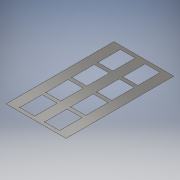
# Autodesk Inventor part: Assembly Stencil
Saved by Autodesk Inventor 2019.4 (Build 234330000, 330)
## iProperties
Created: 2021-01-11
Part Number: Assembly Stencil
Material: Stainless Steel
Document SubType Name: Modeling
Designer: caleb
Density: 8 g/cm^3
Appearance: Semi-Polished
Author: caleb
Autodesk Inventor part; units mm, degrees
ref_plane "YZ Plane" through (0, 0, 0) normal (1, 0, 0) x (0, 1, 0)
ref_plane "XZ Plane" through (0, 0, 0) normal (0, 1, 0) x (-1, 0, 0)
ref_plane "XY Plane" through (0, 0, 0) normal (0, 0, 1) x (1, 0, 0)
sketch "Sketch1" plane through (0, 0, 0) normal (0, 1, 0) x (-1, 0, 0)
  line L0 (-60, 108) -> (60, 108)
  line L1 (60, 108) -> (60, -108)
  line L2 (60, -108) -> (-60, -108)
  line L3 (-60, -108) -> (-60, 108)
  line L4 (-60, 108) -> (60, -108) construction
  line L5 (60, 108) -> (-60, -108) construction
  point P0 (0, 0)
  dimension "d0" = 216
  dimension "d1" = 120
  constraints: 12 end point, 2 midpoint, 2 parallel, 1 horizontal, 1 perpendicular
  measures "d0" distance of L0.end L1.end
  measures "d1" distance of L0.start L0.end
extrude "Extrusion1" add sketch "Sketch1" along normal blind 0.1
sketch "Sketch2" plane through (0, 0.1, 0) normal (0, 1, 0) x (1, 0, 0)
  line L0 (-40, -100.8) -> (-10.2, -100.8)
  line L1 (-10, -100.6) -> (-10, -56)
  line L2 (-10.2, -55.8) -> (-39.8, -55.8)
  line L3 (-40, -56) -> (-40, -100.8)
  line L4 (-60, -108) -> (60, -108) projected
  line L5 (-60, 108) -> (-60, -108) projected
  circle A0 centre (-40, -100.8) radius 1
  arc A1 (-39.8, -55.8) -> (-40, -56) centre (-39.8, -56) ccw
  arc A2 (-10, -56) -> (-10.2, -55.8) centre (-10.2, -56) ccw
  arc A3 (-10.2, -100.8) -> (-10, -100.6) centre (-10.2, -100.6) ccw
  line L6 (-40, -3.8) -> (-40, -48.6)
  arc A4 (-39.8, -3.6) -> (-40, -3.8) centre (-39.8, -3.8) ccw
  circle A5 centre (-40, -48.6) radius 1
  line L7 (-10.2, -3.6) -> (-39.8, -3.6)
  line L8 (-40, -48.6) -> (-10.2, -48.6)
  line L9 (-10, -48.4) -> (-10, -3.8)
  arc A6 (-10, -3.8) -> (-10.2, -3.6) centre (-10.2, -3.8) ccw
  arc A7 (-10.2, -48.6) -> (-10, -48.4) centre (-10.2, -48.4) ccw
  line L10 (-40, 48.4) -> (-40, 3.6)
  arc A8 (-39.8, 48.6) -> (-40, 48.4) centre (-39.8, 48.4) ccw
  circle A9 centre (-40, 3.6) radius 1
  line L11 (-10.2, 48.6) -> (-39.8, 48.6)
  line L12 (-40, 3.6) -> (-10.2, 3.6)
  line L13 (-10, 3.8) -> (-10, 48.4)
  arc A10 (-10, 48.4) -> (-10.2, 48.6) centre (-10.2, 48.4) ccw
  arc A11 (-10.2, 3.6) -> (-10, 3.8) centre (-10.2, 3.8) ccw
  line L14 (-40, 100.6) -> (-40, 55.8)
  arc A12 (-39.8, 100.8) -> (-40, 100.6) centre (-39.8, 100.6) ccw
  circle A13 centre (-40, 55.8) radius 1
  line L15 (-10.2, 100.8) -> (-39.8, 100.8)
  line L16 (-40, 55.8) -> (-10.2, 55.8)
  line L17 (-10, 56) -> (-10, 100.6)
  arc A14 (-10, 100.6) -> (-10.2, 100.8) centre (-10.2, 100.6) ccw
  arc A15 (-10.2, 55.8) -> (-10, 56) centre (-10.2, 56) ccw
  line L18 (10, -56) -> (10, -100.8)
  arc A16 (10.2, -55.8) -> (10, -56) centre (10.2, -56) ccw
  circle A17 centre (10, -100.8) radius 1
  line L19 (39.8, -55.8) -> (10.2, -55.8)
  line L20 (10, -100.8) -> (39.8, -100.8)
  line L21 (40, -100.6) -> (40, -56)
  arc A18 (40, -56) -> (39.8, -55.8) centre (39.8, -56) ccw
  arc A19 (39.8, -100.8) -> (40, -100.6) centre (39.8, -100.6) ccw
  line L22 (10, -3.8) -> (10, -48.6)
  arc A20 (10.2, -3.6) -> (10, -3.8) centre (10.2, -3.8) ccw
  circle A21 centre (10, -48.6) radius 1
  line L23 (39.8, -3.6) -> (10.2, -3.6)
  line L24 (10, -48.6) -> (39.8, -48.6)
  line L25 (40, -48.4) -> (40, -3.8)
  arc A22 (40, -3.8) -> (39.8, -3.6) centre (39.8, -3.8) ccw
  arc A23 (39.8, -48.6) -> (40, -48.4) centre (39.8, -48.4) ccw
  line L26 (10, 48.4) -> (10, 3.6)
  arc A24 (10.2, 48.6) -> (10, 48.4) centre (10.2, 48.4) ccw
  circle A25 centre (10, 3.6) radius 1
  line L27 (39.8, 48.6) -> (10.2, 48.6)
  line L28 (10, 3.6) -> (39.8, 3.6)
  line L29 (40, 3.8) -> (40, 48.4)
  arc A26 (40, 48.4) -> (39.8, 48.6) centre (39.8, 48.4) ccw
  arc A27 (39.8, 3.6) -> (40, 3.8) centre (39.8, 3.8) ccw
  line L30 (10, 100.6) -> (10, 55.8)
  arc A28 (10.2, 100.8) -> (10, 100.6) centre (10.2, 100.6) ccw
  circle A29 centre (10, 55.8) radius 1
  line L31 (39.8, 100.8) -> (10.2, 100.8)
  line L32 (10, 55.8) -> (39.8, 55.8)
  line L33 (40, 56) -> (40, 100.6)
  arc A30 (40, 100.6) -> (39.8, 100.8) centre (39.8, 100.6) ccw
  arc A31 (39.8, 55.8) -> (40, 56) centre (39.8, 56) ccw
  point P0 (0, 0)
  point P1 (-10, -100.8)
  point P2 (-40, -55.8)
  point P3 (-40, -3.6)
  point P4 (-10, -48.6)
  point P5 (-40, 48.6)
  point P6 (-10, 3.6)
  point P7 (-40, 100.8)
  point P8 (-10, 55.8)
  point P9 (10, -55.8)
  point P10 (40, -100.8)
  point P11 (10, -3.6)
  point P12 (40, -48.6)
  point P13 (10, 48.6)
  point P14 (40, 3.6)
  point P15 (10, 100.8)
  point P16 (40, 55.8)
  dimension "d4" = 30
  dimension "d5" = 45
  dimension "d6" = 7.2
  dimension "d7" = 20
  dimension "d8" = 2
  dimension "d9" = 0.2
  dimension "d12" = 52.2
  dimension "d15" = 50
  constraints: 64 end point, 48 point on circle, 32 centre point, 32 point on line, 8 coincident, 6 tangent, 2 equal radius, 2 horizontal, 2 parallel, 1 perpendicular, 1 vertical, 147 other
  measures "d4" distance of L0.start point (-10, -100.8)
  measures "d5" distance of point (-40, -55.8) L0.start
  measures "d6" distance between parallel lines of L4 L0
  measures "d7" distance between parallel lines of L5 L3
  measures "d8" diameter of A0
  measures "d9" radius of A1
  measures "d12" distance of A1.centre A4.centre
  measures "d15" distance of A1.centre A16.centre
extrude "Extrusion2" cut sketch "Sketch2" against normal through all
body "Solid1"
